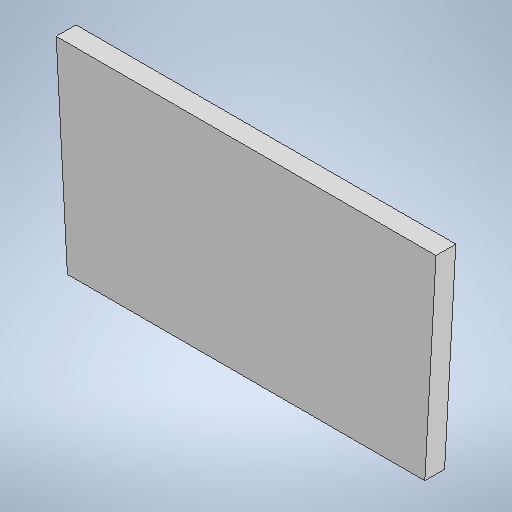
# Autodesk Inventor part: Part5
Saved by Autodesk Inventor 2025.3 (Build 293356000, 356)
## iProperties
Created: 2025-07-05
Part Number: Part5
Material: Generic
Document SubType Name: Modeling
Designer: steve
Density: 1 g/cm^3
Appearance: Default
Author: steve
Autodesk Inventor part; units mm, degrees
ref_plane "YZ Plane" through (0, 0, 0) normal (1, 0, 0) x (0, 1, 0)
ref_plane "XZ Plane" through (0, 0, 0) normal (0, 1, 0) x (-1, 0, 0)
ref_plane "XY Plane" through (0, 0, 0) normal (0, 0, 1) x (1, 0, 0)
sketch "Sketch1" plane through (0, 0, 0) normal (0, 0, 1) x (1, 0, 0)
  line L0 (-18.3788, 14.9409) -> (35.7312, 14.9409)
  line L1 (-20.0738, 45.3109) -> (37.4262, 45.3109)
  line L2 (35.7312, 14.9409) -> (37.4262, 45.3109)
  line L3 (-20.0738, 45.3109) -> (-18.3788, 14.9409)
  line L4 (8.6762, 45.3109) -> (8.6762, 16.4508)
  point P0 (0, 0)
  point P1 (8.6762, 14.9409)
  dimension "d0" = 54.11
  dimension "d1" = 57.5
  dimension "d2" = 30.37
  dimension "d3" = 0
  constraints: 10 end point, 2 horizontal, 2 midpoint, 1 vertical
  measures "d0" distance of L0.start L0.end
  measures "d1" distance of L1.start L1.end
  measures "d2" distance between parallel lines of L1 L0
  measures "d3" horizontal distance of point (8.676, 14.941) L4.start
extrude "Extrusion1" add sketch "Sketch1" along normal blind 3
body "Solid1"
